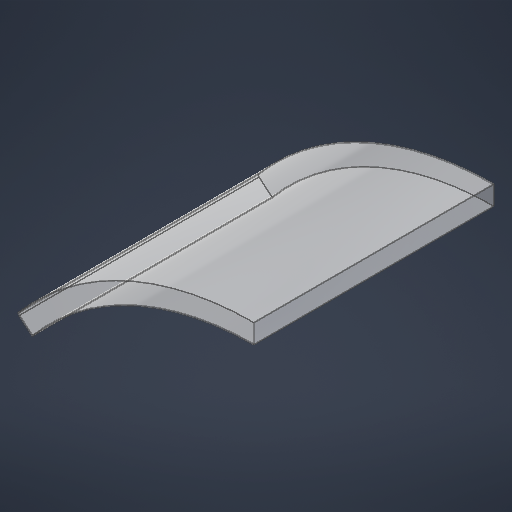
# Autodesk Inventor part: Water Tank
Saved by Autodesk Inventor 2026 (Build 300175000, 175)
## iProperties
Created: 2025-11-05
Part Number: Water Tank
Material: Polycarbonate, Clear
Document SubType Name: Modeling
Designer: Brandon Portillo
Mass: 432308 g
Surface Area: 68365.3 cm^2
Volume: 360257 cm^3
Density: 1.2 g/cm^3
Appearance: Polycarbonate - Clear
Author: Brandon Portillo
Autodesk Inventor part; units mm, degrees
ref_plane "YZ Plane" through (0, 0, 0) normal (1, 0, 0) x (0, 1, 0)
ref_plane "XY Plane" through (0, 0, 0) normal (0, 0, 1) x (1, 0, 0)
sketch "Sketch1" plane through (0, 0, 0) normal (0, 0, 1) x (1, 0, 0)
  arc A0 (0, 2120) -> (-1624.0142, 1362.7097) centre (0, 0) ccw
  line L0 (0, 1985) -> (0, 2120)
  line L1 (0, 0) -> (2120, 0) construction
  line L2 (-1520.5982, 1275.9334) -> (-1624.0142, 1362.7097)
  line L3 (0, 0) -> (2120, 0) construction
  arc A1 (0, 1985) -> (-1520.5982, 1275.9334) centre (0, 0) ccw
  dimension "d0" = 4240
  dimension "d1" = 90
  dimension "d2" = 140
  dimension "d5" = 1985
  constraints: 8 end point, 4 point on circle, 2 centre point, 2 coincident, 2 horizontal, 2 line through centre
  measures "d0" diameter of A0
  measures "d1" angle of L1 L0
  measures "d2" angle of L3 L2
  measures "d5" radius of A1
extrude "Extrusion1" add sketch "Sketch1" along normal blind 1650
ref_plane "Work Plane1" through (-1520.5982, 1275.9334, 0) normal (0, 1, 0) x (0, 0, 1)
fillet "Fillet1" radius 15 1 edges at (-1624.0142, 1362.7097, 825)
shell "Shell2" thickness 4 removed faces 1 at (0, 2030, 550)
body "Solid1"
